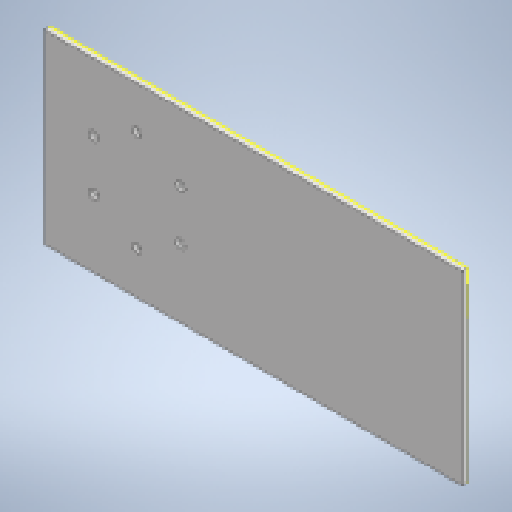
# Autodesk Inventor part: base plate
Saved by Autodesk Inventor 2025 (Build 290162000, 162)
## iProperties
Created: 2025-07-05
Part Number: base plate
Material: 一般
Document SubType Name: Modeling
Designer: gavin
Density: 1 g/cm^3
Appearance: 預設
Author: gavin
Autodesk Inventor part; units mm, degrees
ref_plane "YZ Plane" through (0, 0, 0) normal (1, 0, 0) x (0, 1, 0)
ref_plane "XZ Plane" through (0, 0, 0) normal (0, 1, 0) x (-1, 0, 0)
ref_plane "XY Plane" through (0, 0, 0) normal (0, 0, 1) x (1, 0, 0)
sketch "草圖1" plane through (0, 0, 0) normal (0, 0, 1) x (1, 0, 0)
  circle A0 centre (-46.7654, 27) radius 3.275 construction
  circle A1 centre (46.7654, -27) radius 3.275 construction
  circle A2 centre (-46.7654, -27) radius 3.275 construction
  circle A3 centre (0, 54) radius 3.275 construction
  circle A4 centre (46.7654, 27) radius 3.275 construction
  circle A5 centre (0, -54) radius 3.275 construction
  circle A6 centre (0, 0) radius 60 construction
  circle A7 centre (0, 0) radius 48 construction
  line L0 (350, -100) -> (-100, -100)
  line L1 (-100, -100) -> (-100, 100)
  line L2 (-100, 100) -> (350, 100)
  line L3 (350, 100) -> (350, -100)
  circle A8 centre (0, 54) radius 2.5
  circle A9 centre (-46.7654, 27) radius 2.5
  circle A10 centre (-46.7654, -27) radius 2.5
  circle A11 centre (0, -54) radius 2.5
  circle A12 centre (46.7654, -27) radius 2.5
  circle A13 centre (46.7654, 27) radius 2.5
  dimension "d0" = 450
  dimension "d1" = 200
  dimension "d2" = 100
  dimension "d3" = 100
  dimension "d6" = 5
  dimension "d9" = 360
  constraints: 8 end point, 6 centre point, 2 parallel, 1 coincident, 1 horizontal, 1 perpendicular, 13 other
  measures "d0" distance of L0.start L0.end
  measures "d1" distance of L2.end L0.start
  measures "d2" distance from line of point (0, 0) L1
  measures "d3" distance from line of L2 point (0, 0)
  measures "d6" diameter of A8
extrude "擠出1" add sketch "草圖1" along normal blind 6
chamfer "倒角1" distance 2.5 angle 45 6 edges at (-2.5, -54, 6) (-49.2654, -27, 6) (-49.2654, 27, 6) (-2.5, 54, 6) (44.2654, 27, 6) (44.2654, -27, 6)
sketch "草圖2" plane through (0, 0, 0) normal (0, 0, -1) x (-1, 0, 0)
  line L0 (-350, 100) -> (100, 100) projected
  line L1 (-350, -100) -> (-350, 100) projected
  line L2 (100, -100) -> (-350, -100) projected
  line L3 (100, 100) -> (100, -100) projected
  circle A0 centre (-46.7654, 27) radius 2.5 projected
  circle A1 centre (-46.7654, -27) radius 2.5 projected
  circle A2 centre (0, -54) radius 2.5 projected
  circle A3 centre (46.7654, -27) radius 2.5 projected
  circle A4 centre (46.7654, 27) radius 2.5 projected
  circle A5 centre (0, 54) radius 2.5 projected
  point P0 (0, 0)
